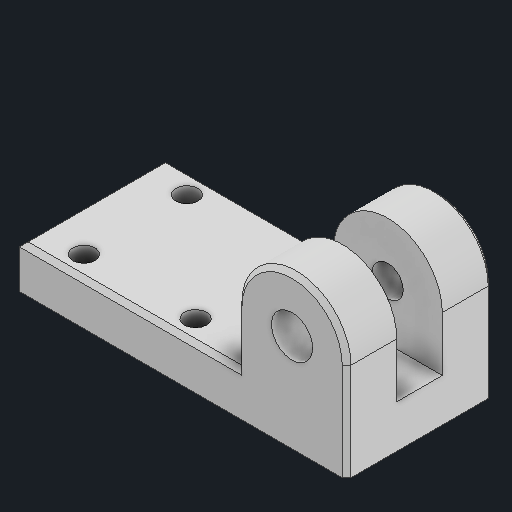
# Autodesk Inventor part: Part3
Saved by Autodesk Inventor 2025.1 (Build 291241020, 241B)
## iProperties
Created: 2025-05-01
Part Number: Part3
Material: Generic
Document SubType Name: Modeling
Designer: Joshua Eah
Density: 1 g/cm^3
Appearance: Default
Author: Joshua Eah
Autodesk Inventor part; units mm, degrees
note: some values were not read from the file. Chosen so that the rebuilt part matches the saved one: direction of "Hole3".
ref_plane "YZ Plane" through (0, 0, 0) normal (1, 0, 0) x (0, 1, 0)
ref_plane "XZ Plane" through (0, 0, 0) normal (0, 1, 0) x (-1, 0, 0)
ref_plane "XY Plane" through (0, 0, 0) normal (0, 0, 1) x (1, 0, 0)
sketch "Sketch1" plane through (0, 0, 0) normal (0, 1, 0) x (-1, 0, 0)
  line L0 (0, 0) -> (38.1, 0)
  line L1 (38.1, 0) -> (38.1, -17)
  line L2 (38.1, -17) -> (0, -17)
  line L3 (0, -17) -> (0, 0)
  circle A0 centre (33.1, -2.5019) radius 1
  circle A1 centre (20.1, -2.5019) radius 1
  circle A2 centre (33.1, -14.5019) radius 1
  circle A3 centre (20.1, -14.5019) radius 1
  dimension "d0" = 38.1
  dimension "d1" = 17
  dimension "d41" = 2
  dimension "d42" = 2
  dimension "d43" = 2
  dimension "d44" = 2
  dimension "d45" = 13
  dimension "d46" = 12
  dimension "d47" = 2.5019
  dimension "d48" = 5
  constraints: 8 end point, 4 centre point, 2 horizontal alignment, 2 parallel, 2 vertical alignment, 1 horizontal, 1 perpendicular
  measures "d0" distance of L1.end L2.end
  measures "d1" distance of L0.end L1.end
  measures "d41" diameter of A0
  measures "d42" diameter of A1
  measures "d43" diameter of A2
  measures "d44" diameter of A3
  measures "d45" distance of A1.centre A0.centre
  measures "d46" distance of A2.centre A0.centre
  measures "d47" distance from line of L0 A0.centre
  measures "d48" distance from line of L1 A0.centre
extrude "Extrusion1" add sketch "Sketch1" along normal blind 5 contours L0 L1 L2 L3 | A0 | A1 | A2 | A3
sketch "Sketch2" plane through (-38.1, 0, 0) normal (0, 0, 1) x (1, 0, 0)
  line L0 (0, 0) -> (38.1, 0) projected
  line L1 (38.1, 0) -> (38.1, 5) projected
  line L2 (0, 5) -> (38.1, 5) projected
  line L3 (0, 0) -> (0, 5) projected
  line L4 (38.1, 5) -> (25.4, 5)
  line L5 (25.4, 5) -> (25.4, 17.7)
  line L6 (25.4, 17.7) -> (38.1, 17.7)
  line L7 (38.1, 17.7) -> (38.1, 5)
  line L8 (31.75, 17.7) -> (31.75, 5) construction
  circle A0 centre (31.75, 11.35) radius 1.5
  point P0 (25.4, 5)
  dimension "d6" = 12.7
  dimension "d7" = 12.7
  dimension "d14" = 3
  constraints: 10 end point, 3 midpoint, 2 parallel, 1 centre point, 1 horizontal, 1 perpendicular
  measures "d6" distance of L5.end L6.end
  measures "d7" distance of L4.end L5.end
  measures "d14" diameter of A0
extrude "Extrusion2" add sketch "Sketch2" against normal up to surface (17 mm away) contours L2 L5 L6 L7 | A0
sketch "Sketch3" plane through (-12.7, 17.7, 0) normal (0, 1, 0) x (1, 0, 0)
  line L0 (12.7, 17) -> (0, 17) projected
  line L1 (0, 0) -> (0, 17) projected
  line L2 (12.7, 0) -> (0, 0) projected
  line L3 (12.7, 0) -> (12.7, 17) projected
  line L4 (0, 8.5) -> (12.7, 8.5) construction
  line L5 (0, 5.85) -> (12.7, 5.85)
  line L6 (12.7, 5.85) -> (12.7, 11.15)
  line L7 (12.7, 11.15) -> (0, 11.15)
  line L8 (0, 11.15) -> (0, 5.85)
  line L9 (0, 5.85) -> (12.7, 11.15) construction
  line L10 (12.7, 5.85) -> (0, 11.15) construction
  point P0 (12.7, 0)
  point P1 (6.35, 8.5)
  point P2 (0, 11.15)
  point P3 (0, 5.85)
  point P4 (12.7, 5.85)
  dimension "d10" = 5.3
  constraints: 14 end point, 5 midpoint, 2 parallel, 1 horizontal, 1 perpendicular, 1 point on line
  measures "d10" distance of L6.end L5.end
extrude "Extrusion3" cut sketch "Sketch3" against normal up to surface (12.7 mm away) contours L3 L5 L1 L7
hole "Hole1" at (-33.1, 0, -2.5019) at (-20.1, 0, -2.5019) at (-20.1, 0, -14.5019) at (-33.1, 0, -14.5019) direction (0, 1, 0) diameter 2.5908 end through all clearance for "Flat Head Machine Screw" size "M2" standard "Ansi Metric M Profile"
fillet "Fillet1" radius 6.35 4 edges at (-12.7, 17.7, -2.925) (0, 17.7, -2.925) (0, 17.7, -14.075) (-12.7, 17.7, -14.075)
chamfer "Chamfer1" distance 0.508 angle 45 9 edges at (-25.4, 5, 0) (-12.7, 8.175, 0) (-10.8402, 15.8402, 0) (0, 5.6751, 0) (-1.8598, 15.8402, -17) (-12.7, 8.175, -17) (0, 5.6751, -17) (-25.4, 5, -17) (-38.1, 5, -8.5)
hole "Hole2" at (-6.35, 11.35, 0) direction (0, 0, -1) diameter 3.6068 end through all clearance for "Flat Head Machine Screw" size "M3" standard "Ansi Metric M Profile"
hole "Hole3" at (-6.35, 11.35, 0) direction (0, 0, -1) diameter 4.8006 depth 5.85 clearance for "Flat Head Machine Screw" size "M4" standard "Ansi Metric M Profile"
body "Solid1"
